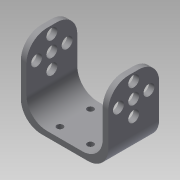
# Autodesk Inventor part: Ufix
Saved by Autodesk Inventor 2014 (Build 180170000, 170)
## iProperties
Created: 2014-03-07
Part Number: Ufix
Material: Générique
Document SubType Name: Modeling
Designer: Grégoire
Density: 1 g/cm^3
Appearance: Par défaut
Author: Grégoire
Autodesk Inventor part; units mm, degrees
ref_plane "YZ Plane" through (0, 0, 0) normal (1, 0, 0) x (0, 1, 0)
ref_plane "XZ Plane" through (0, 0, 0) normal (0, 1, 0) x (-1, 0, 0)
ref_plane "XY Plane" through (0, 0, 0) normal (0, 0, 1) x (1, 0, 0)
sketch "Esquisse1" plane through (0, 0, 0) normal (0, 0, 1) x (1, 0, 0)
  line L0 (0, 0) -> (34.4, 0)
  line L1 (34.4, 0) -> (34.4, 20)
  line L2 (34.4, 20) -> (0, 20)
  line L3 (0, 20) -> (0, 0)
  dimension "d0" = 34.4
  dimension "d1" = 20
  constraints: 8 end point, 2 parallel, 1 horizontal, 1 perpendicular
  measures "d0" distance of L1.end L2.end
  measures "d1" distance of L0.end L1.end
extrude "Extrusion1" add sketch "Esquisse1" along normal blind 2.2
sketch "Esquisse2" plane through (0, 0, 2.2) normal (0, 0, 1) x (1, 0, 0)
  line L0 (0, 0) -> (34.4, 0) projected
  line L1 (34.4, 20) -> (0, 20) projected
  line L2 (0, 20) -> (0, 0) projected
  line L3 (0, 20) -> (2.2, 20)
  line L4 (2.2, 20) -> (2.2, 0)
  line L5 (2.2, 0) -> (0, 0)
  line L6 (0, 0) -> (0, 20)
  line L7 (17.2, 20) -> (17.2, 0) construction
  line L8 (34.4, 20) -> (32.2, 20)
  line L9 (32.2, 20) -> (32.2, 0)
  line L10 (32.2, 0) -> (34.4, 0)
  line L11 (34.4, 0) -> (34.4, 20)
  dimension "d4" = 2.2
  constraints: 18 end point, 3 symmetric about line, 2 midpoint, 2 parallel, 1 horizontal, 1 perpendicular, 1 point on line
  measures "d4" distance between parallel lines of L4 L2
extrude "Extrusion2" add sketch "Esquisse2" along normal blind 27 contours L2 L1 L4 L0 | L9 L1 L11 L0
sketch "Esquisse3" plane through (34.4, 0, 0) normal (1, 0, 0) x (0, 0, -1)
  line L0 (0, 0) -> (0, 20) construction
  line L1 (-29.2, 0) -> (-29.2, 20) construction
  line L2 (-29.2, 10) -> (0, 10) construction
  circle A0 centre (-20.2, 10) radius 2.15
  line L3 (-20.2, 10) -> (-20.2, 15.2246) construction
  circle A1 centre (-14.2, 10) radius 2.15
  circle A2 centre (-26.2, 10) radius 2.15
  circle A3 centre (-20.2, 10) radius 2.15
  circle A4 centre (-20.2, 16) radius 2.15
  circle A5 centre (-20.2, 4) radius 2.15
  circle A6 centre (-20.2, 10) radius 2.15
  dimension "d7" = 9
  dimension "d8" = 4.3
  dimension "d11" = 6
  dimension "d14" = 6
  dimension "d19" = 6
  dimension "d22" = 6
  constraints: 7 centre point, 4 end point, 2 horizontal, 2 midpoint, 2 vertical, 1 perpendicular, 1 point on line, 12 other
  measures "d7" distance of L2.start L3.start
  measures "d8" diameter of A0
  measures "d11" distance of L3.start A1.centre
  measures "d14" distance of L3.start A2.centre
  measures "d19" distance of L3.start A4.centre
  measures "d22" distance of L3.start A5.centre
extrude "Extrusion3" cut sketch "Esquisse3" against normal through all
fillet "Congé1" radius 8 4 edges at (33.3, 20, 29.2) (1.1, 20, 29.2) (1.1, 0, 29.2) (33.3, 0, 29.2)
fillet "Congé2" radius 8 4 edges at (2.2, 10, 2.2) (0, 10, 0) (34.4, 10, 0) (32.2, 10, 2.2)
sketch "Esquisse4" plane through (0, 0, 0) normal (0, 0, -1) x (-1, 0, 0)
  line L0 (-8, 0) -> (-26.4, 0) construction
  line L1 (-26.4, 20) -> (-8.3748, 0) construction
  line L2 (-23.3874, 4) -> (-11.3874, 4) construction
  line L3 (-11.3874, 4) -> (-11.3874, 16) construction
  line L4 (-11.3874, 16) -> (-23.3874, 16) construction
  line L5 (-23.3874, 16) -> (-23.3874, 4) construction
  line L6 (-23.3874, 4) -> (-11.3874, 16) construction
  line L7 (-11.3874, 4) -> (-23.3874, 16) construction
  circle A0 centre (-23.3874, 16) radius 1.25
  line L8 (-17.3874, 16) -> (-17.3874, 4) construction
  line L9 (-23.3874, 10) -> (-11.3874, 10) construction
  circle A1 centre (-11.3874, 16) radius 1.25
  circle A2 centre (-23.3874, 4) radius 1.25
  circle A3 centre (-11.3874, 4) radius 1.25
  point P0 (0, 0)
  point P1 (-17.3874, 10)
  dimension "d29" = 12
  dimension "d30" = 2.5
  constraints: 18 end point, 7 midpoint, 4 centre point, 3 symmetric about line, 2 parallel, 2 perpendicular, 1 coincident, 1 horizontal, 1 point on line, 3 other
  measures "d29" distance of L3.end L4.end
  measures "d30" diameter of A0
extrude "Extrusion4" cut sketch "Esquisse4" against normal through all
equation "\"d2\" = UDepth"
equation "\"d4\" = Depth"
equation "\"d8\" = Holes"
equation "\"d28\" = URound"
equation "\"Depth\" = 2.2"
equation "\"Holes\" = 4.3"
equation "\"UDepth\" = Depth"
equation "\"USize\" = 5"
equation "\"URound\" = 8"
